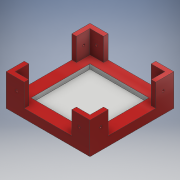
# Autodesk Inventor part: Bottom
Saved by Autodesk Inventor 2018 (Build 220112000, 112)
## iProperties
Created: 2019-10-03
Part Number: Bottom
Material: Generic
Document SubType Name: Modeling
Designer: Ivan
Density: 1 g/cm^3
Appearance: Default
Author: Ivan
Autodesk Inventor part; units mm, degrees
ref_plane "YZ Plane" through (0, 0, 0) normal (1, 0, 0) x (0, 1, 0)
ref_plane "XZ Plane" through (0, 0, 0) normal (0, 1, 0) x (-1, 0, 0)
ref_plane "XY Plane" through (0, 0, 0) normal (0, 0, 1) x (1, 0, 0)
sketch "Sketch2" plane through (0, 0, 0) normal (0, 0, 1) x (1, 0, 0)
  line L0 (-37, 37) -> (37, 37)
  line L1 (37, 37) -> (37, -37)
  line L2 (37, -37) -> (-37, -37)
  line L3 (-37, -37) -> (-37, 37)
  point P0 (0, 0)
  point P1 (0, 37)
  point P2 (37, 0)
  dimension "d0" = 74
  dimension "d1" = 74
  constraints: 8 end point, 2 midpoint, 2 parallel, 1 horizontal, 1 horizontal alignment, 1 perpendicular, 1 vertical alignment
  measures "d0" distance of L0.start L0.end
  measures "d1" distance of L0.end L1.end
extrude "Extrusion1" add sketch "Sketch2" along normal blind 8
sketch "Sketch3" plane through (0, 0, 8) normal (0, 0, 1) x (1, 0, 0)
  line L0 (-37, 37) -> (-21, 37)
  line L1 (-21, 37) -> (-21, 33)
  line L2 (-21, 33) -> (-37, 33)
  line L3 (-37, 33) -> (-37, 37)
  line L4 (-37, 37) -> (-37, -37) construction
  line L5 (37, 37) -> (-37, 37) construction
  line L6 (-37, 33) -> (-33, 33)
  line L7 (-33, 33) -> (-33, 21)
  line L8 (-33, 21) -> (-37, 21)
  line L9 (-37, 21) -> (-37, 33)
  line L10 (21, 33) -> (21, 37)
  line L11 (21, 37) -> (33, 37)
  line L12 (33, 37) -> (33, 33)
  line L13 (33, 33) -> (21, 33)
  line L14 (33, 21) -> (33, 37)
  line L15 (37, 21) -> (33, 21)
  line L16 (37, 37) -> (37, 21)
  line L17 (33, 37) -> (37, 37)
  line L18 (33, -21) -> (37, -21)
  line L19 (37, -21) -> (37, -33)
  line L20 (37, -33) -> (33, -33)
  line L21 (33, -33) -> (33, -21)
  line L22 (21, -33) -> (37, -33)
  line L23 (21, -37) -> (21, -33)
  line L24 (37, -37) -> (21, -37)
  line L25 (37, -33) -> (37, -37)
  line L26 (-21, -33) -> (-21, -37)
  line L27 (-21, -37) -> (-33, -37)
  line L28 (-33, -37) -> (-33, -33)
  line L29 (-33, -33) -> (-21, -33)
  line L30 (-33, -21) -> (-33, -37)
  line L31 (-37, -21) -> (-33, -21)
  line L32 (-37, -37) -> (-37, -21)
  line L33 (-33, -37) -> (-37, -37)
  point P0 (0, 0)
  point P1 (0, 0)
  point P2 (0, 0)
  point P3 (0, 0)
  dimension "d4" = 0
  dimension "d5" = 16
  dimension "d6" = 4
  dimension "d8" = 4
  dimension "d9" = 12
  dimension "d12" = 360
  constraints: 64 end point, 4 parallel, 3 collinear, 2 coincident, 2 horizontal, 2 perpendicular, 66 other
  measures "d4" distance between parallel lines of L4 L3
  measures "d5" distance between parallel lines of L3 L1
  measures "d6" distance of L2.end L0.start
  measures "d8" distance of L6.start L6.end
  measures "d9" distance of L6.end L7.end
extrude "Extrusion2" add sketch "Sketch3" along normal blind 20
sketch "Sketch4" plane through (-37, -37, 0) normal (-1, 0, 0) x (0, 0, 1)
  circle A0 centre (18, 64.5) radius 1
  line L0 (28, 74) -> (28, 58) projected
  line L1 (8, 58) -> (8, 16) projected
  line L2 (0, 37) -> (20, 37) construction
  line L3 (0, 37) -> (20, 37) construction
  circle A1 centre (18, 9.5) radius 1
  line L4 (0, 74) -> (28, 74) projected
  dimension "d16" = 2
  dimension "d18" = 10
  dimension "d19" = 20
  dimension "d20" = 0
  dimension "d26" = 9.5
  constraints: 4 end point, 2 centre point, 2 horizontal, 1 collinear, 1 symmetric about line, 1 other
  measures "d16" diameter of A0
  measures "d18" distance from line of A0.centre L1
  measures "d19" distance of L2.start L2.end
  measures "d20" distance between parallel lines of L2 L3
  measures "d26" distance from line of L4 A0.centre
extrude "Extrusion3" cut sketch "Sketch4" against normal up to surface (4 mm away)
pattern_circular "Circular Pattern1" count 4 over 360 about axis through (0, 0, -10) along (0, 0, 1) of "Extrusion3"
sketch "Sketch5" plane through (0, 0, 8) normal (0, 0, 1) x (1, 0, 0)
  line L0 (-26, -26) -> (26, -26)
  line L1 (26, -26) -> (26, 26)
  line L2 (26, 26) -> (-26, 26)
  line L3 (-26, 26) -> (-26, -26)
  line L4 (-21, -37) -> (21, -37) projected
  line L5 (-37, 21) -> (-37, -21) projected
  point P0 (0, 0)
  point P1 (-26, 0)
  point P2 (0, 26)
  dimension "d27" = 11
  dimension "d28" = 11
  constraints: 8 end point, 2 midpoint, 2 parallel, 1 horizontal, 1 horizontal alignment, 1 perpendicular, 1 vertical alignment
  measures "d27" distance between parallel lines of L4 L0
  measures "d28" distance between parallel lines of L5 L3
extrude "Extrusion4" cut sketch "Sketch5" against normal blind 4
sketch "Sketch6" plane through (-37, 37, 0) normal (0, 1, 0) x (1, 0, 0)
  line L0 (64, -6) -> (64, -3) construction
  line L1 (66.25, -3.75) -> (64, -6) construction
  line L2 (66.25, -3.75) -> (64, -6)
  line L3 (64, -6) -> (64, -3)
  line L4 (64, -3) -> (64, 0)
  line L5 (64.75, -2.25) -> (67, 0) construction
  line L6 (66.25, -3.75) -> (64.75, -2.25)
  line L7 (67, 0) -> (64.75, -2.25)
  line L8 (64, 0) -> (67, 0)
  constraints: 18 end point, 2 collinear, 2 perpendicular, 2 vertical
extrude "Extrusion5" cut sketch "Sketch6" against normal up to surface (63 mm away)
mirror "Mirror1" about plane through (0, 0, 0) normal (1, 0, 0) of "Extrusion5"
sketch "Sketch7" plane through (-37, -37, 0) normal (-1, 0, 0) x (0, 0, 1)
  line L0 (6, 6) -> (3, 6) construction
  line L1 (6, 6) -> (3, 6)
  line L2 (3, 6) -> (0, 6)
  line L3 (3.75, 3.75) -> (6, 6) construction
  line L4 (3.75, 3.75) -> (6, 6)
  line L5 (2.25, 5.25) -> (0, 3) construction
  line L6 (3.75, 3.75) -> (2.25, 5.25)
  line L7 (0, 3) -> (2.25, 5.25)
  line L8 (0, 6) -> (0, 3)
  line L9 (0, 0) -> (28, 0) projected
  point P0 (0, 37)
  point P1 (0, 11)
  dimension "d42" = 6
  dimension "d45" = 3
  dimension "d46" = 5
  constraints: 18 end point, 1 collinear
  measures "d42" distance of L2.end L0.start
  measures "d45" distance of L5.end L2.end
  measures "d46" distance of point (0, 11) L2.end
extrude "Extrusion6" cut sketch "Sketch7" against normal blind 67
equation "\"d1\" = d0"
equation "\"d8\" = d6"
equation "\"d9\" = d5 - d6"
body "Solid1"
